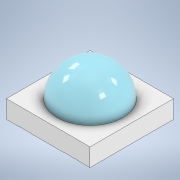
# Autodesk Inventor part: IN-3531SCUV
Saved by Autodesk Inventor 2020.2 (Build 242310000, 310)
## iProperties
Created: 2020-06-16
Part Number: IN-3531SCUV
Material: Generisch
Document SubType Name: Modeling
Designer: Daniel.Kampert
Density: 1 g/cm^3
Appearance: Vorgabe
Author: Daniel.Kampert
Autodesk Inventor part; units mm, degrees
ref_plane "YZ Plane" through (0, 0, 0) normal (1, 0, 0) x (0, 1, 0)
ref_plane "XZ Plane" through (0, 0, 0) normal (0, 1, 0) x (-1, 0, 0)
ref_plane "XY Plane" through (0, 0, 0) normal (0, 0, 1) x (1, 0, 0)
sketch "Skizze3" plane through (0, 0, 0) normal (0, 1, 0) x (-1, 0, 0)
  line L0 (1.65, -1.65) -> (-1.65, -1.65)
  line L1 (-1.65, -1.65) -> (-1.65, 1.65)
  line L2 (-1.65, 1.65) -> (1.65, 1.65)
  line L3 (1.65, 1.65) -> (1.65, -1.65)
  line L4 (1.65, -1.65) -> (-1.65, 1.65) construction
  line L5 (-1.65, -1.65) -> (1.65, 1.65) construction
  point P0 (0, 0)
  dimension "d5" = 3.3
  dimension "d6" = 3.3
  constraints: 12 end point, 2 midpoint, 2 parallel, 1 horizontal, 1 perpendicular
  measures "d5" distance of L1.end L2.end
  measures "d6" distance of L0.end L1.end
extrude "Extrusion2" add sketch "Skizze3" along normal blind 0.7
sketch "Skizze5" plane through (0, 0, 0) normal (0, -1, 0) x (1, 0, 0)
  line L0 (1.65, -1.65) -> (-1.65, -1.65) projected
  line L1 (1.65, 1.65) -> (1.65, -1.65) projected
  line L2 (-1.65, 1.65) -> (1.65, 1.65) projected
  line L3 (-1.65, -1.65) -> (-1.65, 1.65) projected
  line L4 (-0.65, -1.65) -> (0.65, -1.65)
  line L5 (0.65, -1.65) -> (0.65, 1.65)
  line L6 (0.65, 1.65) -> (-0.65, 1.65)
  line L7 (-0.65, 1.65) -> (-0.65, -1.65)
  line L8 (-0.65, -1.65) -> (0.65, 1.65) construction
  line L9 (0.65, -1.65) -> (-0.65, 1.65) construction
  line L10 (-1.65, 0) -> (1.65, 0) construction
  line L11 (1.15, 1.65) -> (1.65, 1.65)
  line L12 (1.65, 1.65) -> (1.65, -1.65)
  line L13 (1.65, -1.65) -> (1.15, -1.65)
  line L14 (1.15, -1.65) -> (1.15, 1.65)
  line L15 (1.15, 1.65) -> (1.65, -1.65) construction
  line L16 (1.65, 1.65) -> (1.15, -1.65) construction
  line L17 (-1.65, 1.65) -> (-1.15, 1.65)
  line L18 (-1.15, -1.65) -> (-1.65, -1.65)
  line L19 (-1.65, -1.65) -> (-1.65, 1.65)
  line L20 (-1.65, 1.65) -> (-1.15, -1.65) construction
  line L21 (-1.15, 1.65) -> (-1.65, -1.65) construction
  line L22 (-1.15, 0.25) -> (-1.2, 0.25)
  line L23 (-1.2, 0.25) -> (-1.2, -0.25)
  line L24 (-1.2, -0.25) -> (-1.15, -0.25)
  line L25 (-1.15, 1.65) -> (-1.15, 0.25)
  line L26 (-1.15, -0.25) -> (-1.15, -1.65)
  point P0 (0, 0)
  point P1 (1.4, 0)
  point P2 (-1.4, 0)
  dimension "d13" = 1.3
  dimension "d14" = 3.3
  dimension "d15" = 0.5
  dimension "d16" = 3.3
  dimension "d19" = 1.4
  dimension "d20" = 0.5
  dimension "d21" = 3.3
  dimension "d22" = 1.4
  dimension "d26" = 0.5
  dimension "d27" = 0.05
  dimension "d28" = 1.4
  constraints: 46 end point, 8 midpoint, 8 parallel, 6 perpendicular, 4 horizontal, 2 point on line, 1 other
  measures "d13" distance of L6.end L5.end
  measures "d14" distance of L5.end L4.end
  measures "d15" distance of L12.end L13.end
  measures "d16" distance of L11.end L12.end
  measures "d19" distance of point (1.4, 0) point (0, 0)
  measures "d20" distance of L18.start L18.end
  measures "d21" distance of L17.end L18.start
  measures "d22" distance of point (0, 0) point (-1.4, 0)
  measures "d26" distance of L22.end L23.end
  measures "d27" distance of L23.end L24.end
  measures "d28" distance of L24.end L18.start
sketch "Skizze4" plane through (0, 0.7, 0) normal (0, 1, 0) x (1, 0, 0)
  line L0 (1.65, 1.65) -> (-1.65, 1.65) projected
  circle A0 centre (0, 0) radius 1.3
  dimension "d9" = 2.6
  constraints: 1 centre point, 1 coincident
  measures "d9" diameter of A0
extrude "Extrusion3" add sketch "Skizze4" along normal blind 1.3
fillet "Rundung1" radius 1.3 1 edges at (-1.3, 2, 0)
extrude "Extrusion5" add sketch "Skizze5" along normal blind 0.01 contours L0 L14 L2 L1 | L0 L7 L2 L5 | L0 L3 L2 L25 L22 L23 L24 L26
